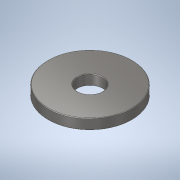
# Autodesk Inventor part: 00-05-002-MetalDisk
Saved by Autodesk Inventor 2022 (Build 260153000, 153)
## iProperties
Created: 2019-05-31
Part Number: 00-05-002-MetalDisk
Material: Edelstahl
Document SubType Name: Modeling
Designer: denni
Density: 8 g/cm^3
Appearance: Halbpoliert
Author: denni
Autodesk Inventor part; units mm, degrees
ref_plane "YZ Plane" through (0, 0, 0) normal (1, 0, 0) x (0, 1, 0)
ref_plane "XZ Plane" through (0, 0, 0) normal (0, 1, 0) x (-1, 0, 0)
ref_plane "XY Plane" through (0, 0, 0) normal (0, 0, 1) x (1, 0, 0)
sketch "Skizze1" plane through (0, 0, 0) normal (0, 0, 1) x (1, 0, 0)
  circle A0 centre (0, 0) radius 7.5
  circle A1 centre (0, 0) radius 2.225
  dimension "d0" = 15
  dimension "d1" = 4.45
  constraints: 2 centre point, 2 coincident
  measures "d0" diameter of A0
  measures "d1" diameter of A1
extrude "Extrusion1" add sketch "Skizze1" along normal blind 1.84
fillet "Rundung1" radius 0.1 4 edges at (-2.225, 0, 0) (-2.225, 0, 1.84) (-7.5, 0, 0) (-7.5, 0, 1.84)
